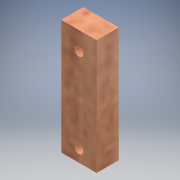
# Autodesk Inventor part: 支架 assembly
Saved by Autodesk Inventor 2017 (Build 210142000, 142)
## iProperties
Created: 2019-12-03
Part Number: 支架 assembly
Material: Generic
Document SubType Name: Modeling
Designer: User
Density: 1 g/cm^3
Appearance: Default
Author: User
Autodesk Inventor part; units mm, degrees
ref_plane "YZ Plane" through (0, 0, 0) normal (1, 0, 0) x (0, 1, 0)
ref_plane "XZ Plane" through (0, 0, 0) normal (0, 1, 0) x (-1, 0, 0)
ref_plane "XY Plane" through (0, 0, 0) normal (0, 0, 1) x (1, 0, 0)
sketch "Sketch1" plane through (0, 0, 0) normal (0, 0, 1) x (1, 0, 0)
  line L0 (-4, 2.5) -> (4, 2.5)
  line L1 (4, 2.5) -> (4, -2.5)
  line L2 (4, -2.5) -> (-4, -2.5)
  line L3 (-4, -2.5) -> (-4, 2.5)
  line L4 (-4, 2.5) -> (4, -2.5) construction
  line L5 (4, 2.5) -> (-4, -2.5) construction
  point P0 (0, 0)
  dimension "d0" = 8
  dimension "d1" = 5
  constraints: 12 end point, 2 midpoint, 2 parallel, 1 horizontal, 1 perpendicular
  measures "d0" distance of L1.end L2.end
  measures "d1" distance of L0.end L1.end
extrude "Extrusion1" add sketch "Sketch1" along normal blind 25
sketch "Sketch2" plane through (-4, -2.5, 0) normal (0, -1, 0) x (1, 0, 0)
  circle A0 centre (4, 1.7) radius 1
  circle A1 centre (4, 20.8) radius 1
  point P0 (4, 0)
  dimension "d4" = 2
  dimension "d5" = 2
  constraints: 2 centre point
  measures "d4" diameter of A0
  measures "d5" diameter of A1
extrude "Extrusion2" cut sketch "Sketch2" against normal up to next
sketch "Sketch3" plane through (0, 0, 0) normal (0, 0, -1) x (-1, 0, 0)
  line L0 (-4, -2.5) -> (4, -2.5) projected
  line L1 (-4, -2.5) -> (-4, 2.5) projected
  line L2 (4, -2.5) -> (-4, -2.5)
  line L3 (-4, -2.5) -> (-4, 2.5)
  line L4 (-4, 2.5) -> (4, 2.5)
  line L5 (4, 2.5) -> (4, -2.5)
  point P0 (0, 0)
  constraints: 8 end point, 2 parallel, 1 horizontal, 1 perpendicular
extrude "Extrusion3" add sketch "Sketch3" along normal blind 1
body "Solid1"
